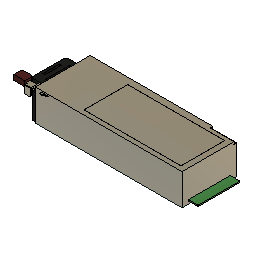
HPE flex psu (Autodesk Fusion 360 design; units mm, degrees)
Autodesk Fusion 360 part; units mm, degrees
sketch "Sketch1" plane through (0, 0, 0) normal (0, 0, 1) x (1, 0, 0)
  line L0 (-91.5, -34.15) -> (91.5, -34.15)
  line L1 (91.5, -34.15) -> (91.5, 34.15)
  line L2 (91.5, 34.15) -> (-91.5, 34.15)
  line L3 (-91.5, 34.15) -> (-91.5, -34.15)
  line L4 (-91.5, -34.15) -> (91.5, 34.15) construction
  line L5 (91.5, -34.15) -> (-91.5, 34.15) construction
  dimension "d1" = 183
  dimension "d2" = 68.3
  constraint horizontal L0
  constraint perpendicular L0 L1
  constraint parallel L0 L2
  constraint parallel L1 L3
  constraint coincident L4 origin
  constraint coincident L5 origin
  measures "d1" distance of L1.end L2.end
  measures "d2" distance of L0.end L1.end
extrude "Extrude1" add sketch "Sketch1" along normal blind 39.1 makes body 1
sketch "Sketch2" plane through (0, 0, 0) normal (0, 0, -1) x (1, 0, 0)
  line L0 (-91.5, 34.15) -> (-91.5, -34.15)
  line L1 (-91.5, -34.15) -> (91.5, -34.15)
  line L2 (91.5, -34.15) -> (91.5, 34.15)
  line L3 (91.5, 34.15) -> (-91.5, 34.15)
sketch "Sketch3" plane through (0, 34.15, 0) normal (0, 1, 0) x (-1, 0, 0)
  line L0 (-91.5, 0) -> (91.5, 0)
  line L1 (91.5, 0) -> (91.5, 39.1)
  line L2 (91.5, 39.1) -> (-91.5, 39.1)
  line L3 (-91.5, 39.1) -> (-91.5, 0)
  line L4 (91.5, 0) -> (91.5, 39.1)
  line L5 (61.5, 22.2) -> (121.5, 22.2)
  line L6 (121.5, 22.2) -> (121.5, 16.9)
  line L7 (121.5, 16.9) -> (61.5, 16.9)
  line L8 (61.5, 16.9) -> (61.5, 22.2)
  line L9 (61.5, 22.2) -> (121.5, 16.9) construction
  line L10 (121.5, 22.2) -> (61.5, 16.9) construction
  line L11 (82.2, 25.55) -> (100.8, 25.55)
  line L12 (100.8, 25.55) -> (100.8, 13.55)
  line L13 (100.8, 13.55) -> (82.2, 13.55)
  line L14 (82.2, 13.55) -> (82.2, 25.55)
  line L15 (82.2, 25.55) -> (100.8, 13.55) construction
  line L16 (100.8, 25.55) -> (82.2, 13.55) construction
  point P0 (91.5, 19.55)
  point P1 (91.5, 19.55)
  dimension "d5" = 60
  dimension "d6" = 5.3
  dimension "d7" = 18.6
  dimension "d8" = 12
  constraint coincident L0.end L1.start
  constraint coincident L1.end L2.start
  constraint horizontal L5
  constraint perpendicular L5 L6
  constraint parallel L5 L7
  constraint parallel L6 L8
  constraint coincident L9 P1
  constraint coincident L10 P1
  constraint midpoint L1 P1
  constraint horizontal L11
  constraint perpendicular L11 L12
  constraint parallel L11 L13
  constraint parallel L12 L14
  constraint coincident L15 P1
  constraint coincident L16 P1
  constraint coincident P1 P0
  measures "d5" distance of L6.end L7.end
  measures "d6" distance of L5.end L6.end
  measures "d7" distance of L12.end L13.end
  measures "d8" distance of L11.end L12.end
extrude "Extrude2" add sketch "Sketch3" against normal blind 43.7 contours L1 L4 L7 L12 L13 | L1 L4 L5 L7 L12 | L1 L4 L5 L11 L12 | L5 L6 L7 L12 bodies 1
sketch "Sketch4" plane through (0, 0, 16.9) normal (0, 0, -1) x (1, 0, 0)
  line L0 (-121.5, -34.15) -> (-100.8, -34.15)
  line L1 (-100.8, -34.15) -> (-100.8, 9.55)
  line L2 (-100.8, 9.55) -> (-121.5, 9.55)
  line L3 (-121.5, 9.55) -> (-121.5, -34.15)
  line L4 (-121.5, 9.55) -> (-100.8, 9.55)
  line L5 (-100.8, 9.55) -> (-100.8, -34.15)
  line L6 (-100.8, -34.15) -> (-121.5, -34.15)
  line L7 (-121.5, -34.15) -> (-121.5, 9.55)
  line L8 (-121.5, -7) -> (-110.5, -7)
  line L9 (-106.7103, 9.55) -> (-106.7103, 9)
  line L10 (-106.7103, 9) -> (-106.7103, 2.7)
  line L11 (-106.7103, 2.7) -> (-121.5, 2.7)
  line L12 (-110.5, -7) -> (-110.5, 2.7)
  line L13 (-106.7103, 2.7) -> (-86, 2.7)
  line L14 (-110.5, -7) -> (-110.5, -34.15)
  line L15 (-110.5, -34.15) -> (-110.5, -27.85)
  line L16 (-110.5, -27.85) -> (-100.8, -27.85)
  line L17 (-100.8, 2.7) -> (-100.8, -27.85)
  dimension "d11" = 11
  dimension "d12" = 6.3
  dimension "d13" = 6.3
  constraint horizontal L4
  constraint vertical L5
  constraint horizontal L6
  constraint vertical L7
  constraint coincident L0.end L1.start
  constraint coincident L2.end L3.start
  constraint coincident L3 L8.start
  constraint perpendicular L3 L8
  constraint coincident L2 L9.start
  constraint perpendicular L2 L9
  constraint perpendicular L4 L10
  constraint coincident L7 L11.end
  constraint perpendicular L7 L11
  constraint coincident L11 L12.end
  constraint perpendicular L11 L12
  constraint perpendicular L10 L13
  constraint coincident L6 L14.end
  constraint perpendicular L6 L14
  constraint parallel L14 L15
  constraint coincident L1 L16.end
  constraint perpendicular L1 L16
  constraint coincident L13 L17.start
  constraint coincident L5 L17.start
  measures "d11" distance of L8.start L8.end
  measures "d12" distance of L9.end L10.end
  measures "d13" distance of L14.end L15.end
extrude "Extrude3" cut sketch "Sketch4" against normal blind 45 contours L1 L5 L11 L12 L13 L14 L16 L17 bodies 1
sketch "Sketch5" plane through (0, 0, 13.55) normal (0, 0, -1) x (1, 0, 0)
  line L0 (-100.8, -34.15) -> (-91.5, -34.15)
  line L1 (-91.5, -34.15) -> (-91.5, 9.55)
  line L2 (-91.5, 9.55) -> (-100.8, 9.55)
  line L3 (-100.8, 9.55) -> (-100.8, -34.15)
  line L4 (-100.8, 9.55) -> (-91.5, -34.15)
  line L5 (-100.8, 5.2) -> (-91.5, 5.2)
  line L6 (-91.5, 5.2) -> (-91.5, -29.8)
  line L7 (-91.5, -29.8) -> (-100.8, -29.8)
  line L8 (-100.8, -29.8) -> (-100.8, 5.2)
  line L9 (-100.8, 5.2) -> (-91.5, -29.8) construction
  line L10 (-91.5, 5.2) -> (-100.8, -29.8) construction
  point P0 (-96.15, -12.3)
  dimension "d16" = 35
  constraint coincident L2.end L3.start
  constraint coincident L0.end L1.start
  constraint horizontal L5
  constraint perpendicular L5 L6
  constraint parallel L5 L7
  constraint parallel L6 L8
  constraint coincident L9 P0
  constraint coincident L10 P0
  constraint coincident L3 L5.start
  constraint midpoint L4 P0
  measures "d16" distance of L5.end L6.end
extrude "Extrude4" cut sketch "Sketch5" against normal blind 35 contours L3 L4 L5 L7 L8 | L1 L4 L5 L6 L7 bodies 1
sketch "Sketch6" plane through (0, 0, 16.9) normal (0, 0, -1) x (1, 0, 0)
  line L0 (-110.5, 2.7) -> (-100.8, 2.7)
  line L1 (-100.8, 2.7) -> (-100.8, 5.2)
  line L2 (-100.8, 5.2) -> (-100.8, 9.55)
  line L3 (-100.8, 9.55) -> (-121.5, 9.55)
  line L4 (-121.5, 9.55) -> (-121.5, -34.15)
  line L5 (-121.5, -34.15) -> (-100.8, -34.15)
  line L6 (-100.8, -34.15) -> (-100.8, -29.8)
  line L7 (-100.8, -29.8) -> (-100.8, -27.85)
  line L8 (-100.8, -27.85) -> (-110.5, -27.85)
  line L9 (-110.5, -27.85) -> (-110.5, 2.7)
  line L10 (-121.5, -2.463) -> (-118.3, -2.463)
  line L11 (-118.3, -2.463) -> (-118.3, -34.15)
  line L12 (-118.3, -2.463) -> (-118.3, 9.55)
  line L13 (-118.3, 9.55) -> (-118.3, -2.05)
  line L14 (-118.3, -34.15) -> (-118.3, -22.55)
  line L15 (-118.3, -2.05) -> (-115.7, -2.05)
  line L16 (-115.7, -2.05) -> (-118.3, -2.05)
  line L17 (-118.3, -2.05) -> (-118.3, -22.55)
  line L18 (-118.3, -22.55) -> (-115.7, -22.55)
  line L19 (-115.7, -22.55) -> (-115.7, -2.05)
  dimension "d19" = 3.2
  dimension "d20" = 11.6
  dimension "d21" = 11.6
  dimension "d22" = 2.6
  constraint coincident L4 L10.start
  constraint perpendicular L4 L10
  constraint coincident L5 L11.end
  constraint perpendicular L5 L11
  constraint coincident L3 L12.end
  constraint perpendicular L3 L12
  constraint perpendicular L3 L13
  constraint coincident L11 L14.end
  constraint perpendicular L13 L15
  constraint horizontal L16
  constraint vertical L17
  constraint horizontal L18
  constraint vertical L19
  measures "d19" distance of L10.start L10.end
  measures "d20" distance of L12.end L13.end
  measures "d21" distance of L11.end L14.end
  measures "d22" distance of L13.end L15.end
extrude "Extrude5" cut sketch "Sketch6" against normal blind 52 contours L11 L12 L15 L16 L17 L18 L19 bodies 1
sketch "Sketch7" plane through (-91.5, 0, 0) normal (-1, 0, 0) x (0, -1, 0)
  line L0 (-29.8, 13.55) -> (-34.15, 13.55)
  line L1 (-34.15, 13.55) -> (-34.15, 0)
  line L2 (-34.15, 0) -> (34.15, 0)
  line L3 (34.15, 0) -> (34.15, 39.1)
  line L4 (34.15, 39.1) -> (-34.15, 39.1)
  line L5 (-34.15, 39.1) -> (-34.15, 25.55)
  line L6 (-34.15, 25.55) -> (-29.8, 25.55)
  line L7 (-29.8, 25.55) -> (-29.8, 13.55)
  line L8 (5.2, 13.55) -> (5.2, 25.55)
  line L9 (5.2, 25.55) -> (9.55, 25.55)
  line L10 (9.55, 25.55) -> (9.55, 13.55)
  line L11 (9.55, 13.55) -> (5.2, 13.55)
  line L12 (34.15, 0) -> (34.15, 1.5)
  line L13 (34.15, 1.5) -> (10.35, 1.5)
  line L14 (10.35, 1.5) -> (10.35, 32.7)
  line L15 (10.35, 32.7) -> (34.15, 32.7)
  line L16 (34.15, 32.7) -> (34.15, 1.5)
  dimension "d25" = 1.5
  dimension "d26" = 23.8
  dimension "d27" = 31.2
  constraint coincident L2.end L3.start
  constraint perpendicular L2 L12
  constraint horizontal L13
  constraint vertical L14
  constraint horizontal L15
  constraint vertical L16
  measures "d25" distance of L2.end L12.end
  measures "d26" distance of L12.end L13.end
  measures "d27" distance of L12.end L15.end
extrude "Extrude6" add sketch "Sketch7" along normal blind 3.7 separate body contours L3 L13 L14 L15 L16 makes body 2
sketch "Sketch8" plane through (91.5, 0, 0) normal (1, 0, 0) x (0, 1, 0)
  line L0 (-34.15, 0) -> (34.15, 0)
  line L1 (34.15, 0) -> (34.15, 39.1)
  line L2 (34.15, 39.1) -> (-34.15, 39.1)
  line L3 (-34.15, 39.1) -> (-34.15, 0)
  line L4 (-34.15, 0) -> (34.15, 0)
  line L5 (34.15, 0) -> (34.15, 3.4)
  line L6 (34.15, 3.4) -> (-34.15, 3.4)
  line L7 (-34.15, 3.4) -> (-34.15, 0)
  line L8 (34.15, 3.4) -> (-34.15, 3.4)
  line L9 (-34.15, 3.4) -> (-34.15, 4.9)
  line L10 (-34.15, 4.9) -> (34.15, 4.9)
  line L11 (34.15, 4.9) -> (34.15, 3.4)
  line L12 (26.1, 3.4) -> (-26.1, 3.4)
  line L13 (-26.1, 3.4) -> (-26.1, 6.4)
  line L14 (-26.1, 6.4) -> (26.1, 6.4)
  line L15 (26.1, 6.4) -> (26.1, 3.4)
  line L16 (26.1, 3.4) -> (-26.1, 6.4) construction
  line L17 (-26.1, 3.4) -> (26.1, 6.4) construction
  point P0 (0, 4.9)
  dimension "d30" = 3.4
  dimension "d31" = 1.5
  dimension "d32" = 52.2
  constraint horizontal L4
  constraint vertical L5
  constraint horizontal L6
  constraint vertical L7
  constraint coincident L0.start L3.end
  constraint horizontal L8
  constraint vertical L9
  constraint horizontal L10
  constraint vertical L11
  constraint coincident L3 L9.end
  constraint horizontal L12
  constraint perpendicular L12 L13
  constraint parallel L12 L14
  constraint parallel L13 L15
  constraint coincident L16 P0
  constraint coincident L17 P0
  constraint coincident L6 L12.start
  constraint midpoint L10 P0
  measures "d30" distance of L0.start L6.end
  measures "d31" distance of L5.end L10.end
  measures "d32" distance of L13.end L14.end
extrude "Extrude7" add sketch "Sketch8" along normal blind 12 contours L6 L8 L10 L12 L13 L15 bodies 1
sketch "Sketch9" plane through (91.5, 0, 0) normal (1, 0, 0) x (0, 1, 0)
  line L0 (-26.1, 4.9) -> (26.1, 4.9)
  line L1 (26.1, 4.9) -> (26.1, 3.4)
  line L2 (26.1, 3.4) -> (-26.1, 3.4)
  line L3 (-26.1, 3.4) -> (-26.1, 4.9)
  line L4 (-34.15, 0) -> (34.15, 0)
  line L5 (34.15, 0) -> (34.15, 39.1)
  line L6 (34.15, 39.1) -> (-34.15, 39.1)
  line L7 (-34.15, 39.1) -> (-34.15, 0)
  line L8 (-34.15, 39.1) -> (-30.75, 39.1)
  line L9 (-30.75, 39.1) -> (-30.75, 36.1)
  line L10 (-30.75, 36.1) -> (-34.15, 36.1)
  line L11 (-34.15, 36.1) -> (-34.15, 39.1)
  dimension "d35" = 3.4
  dimension "d36" = 3
  constraint horizontal L8
  constraint vertical L9
  constraint horizontal L10
  constraint vertical L11
  constraint coincident L6.end L7.start
  measures "d35" distance of L6.end L8.end
  measures "d36" distance of L6.end L10.end
extrude "Extrude8" cut sketch "Sketch9" against normal blind 29.7 contours L6 L7 L8 L9 L10 L11 bodies 1
sketch "Sketch10" plane through (0, -34.15, 0) normal (0, -1, 0) x (1, 0, 0)
  line L0 (61.8, 36.1) -> (61.8, 39.1)
  line L1 (61.8, 39.1) -> (-91.5, 39.1)
  line L2 (-91.5, 39.1) -> (-91.5, 0)
  line L3 (-91.5, 0) -> (91.5, 0)
  line L4 (91.5, 0) -> (91.5, 36.1)
  line L5 (91.5, 36.1) -> (61.8, 36.1)
  line L6 (-91.5, 39.1) -> (-84.1, 39.1)
  line L7 (-84.1, 39.1) -> (-74.1, 39.1)
  line L8 (-84.1, 39.1) -> (-74.1, 39.1)
  line L9 (-74.1, 39.1) -> (-74.1, 36.3)
  line L10 (-74.1, 36.3) -> (-84.1, 36.3)
  line L11 (-84.1, 36.3) -> (-84.1, 39.1)
  line L12 (-74.1, 39.1) -> (-74.5, 39.1)
  line L13 (-74.1, 39.1) -> (-75.4, 39.1)
  line L14 (-75.4, 39.1) -> (-75.4, 36.5)
  line L15 (-75.4, 36.5) -> (-75.4, 36.3)
  line L16 (-75.4, 39.1) -> (-75.4, 37.4)
  line L17 (-75.4, 37.4) -> (-75.4, 36.4)
  line L18 (-75.4, 37.4) -> (-84.1, 37.4)
  line L19 (-84.1, 37.4) -> (-84.1, 36.4)
  line L20 (-84.1, 36.4) -> (-75.4, 36.4)
  line L21 (-75.4, 36.4) -> (-75.4, 37.4)
  dimension "d39" = 7.4
  dimension "d40" = 10
  dimension "d41" = 10
  dimension "d42" = 2.8
  dimension "d43" = 1.3
  dimension "d44" = 1.7
  dimension "d45" = 1
  dimension "d46" = 1
  constraint coincident L1.end L2.start
  constraint perpendicular L2 L6
  constraint perpendicular L2 L7
  constraint horizontal L8
  constraint vertical L9
  constraint horizontal L10
  constraint vertical L11
  constraint coincident L7 L12.end
  constraint perpendicular L9 L13
  constraint perpendicular L13 L14
  constraint coincident L10 L15.end
  constraint perpendicular L10 L15
  constraint perpendicular L13 L16
  constraint perpendicular L13 L17
  constraint horizontal L18
  constraint vertical L19
  constraint horizontal L20
  constraint vertical L21
  constraint coincident L11 L19.end
  measures "d39" distance of L1.end L6.end
  measures "d40" distance of L6.end L7.end
  measures "d41" distance of L6.end L7.end
  measures "d42" distance of L6.end L10.end
  measures "d43" distance of L7.end L13.end
  measures "d44" distance of L13.end L16.end
  measures "d45" distance of L16.end L17.end
  measures "d46" distance of L16.end L17.end
extrude "Extrude9" add sketch "Sketch10" along normal blind 2.2 contours L11 L14 L15 L17 L18 L19 L20 L21 bodies 1
sketch "Sketch11" plane through (0, 0, 37.4) normal (0, 0, 1) x (-1, 0, 0)
  line L0 (75.4, 34.15) -> (84.1, 34.15)
  line L1 (84.1, 34.15) -> (84.1, 36.35)
  line L2 (84.1, 36.35) -> (75.4, 36.35)
  line L3 (75.4, 36.35) -> (75.4, 34.15)
  line L4 (84.1, 36.35) -> (81.7, 36.35)
  line L5 (81.7, 36.35) -> (75.4, 34.15)
  dimension "d49" = 2.4
  constraint coincident L1.end L2.start
  constraint perpendicular L1 L4
  constraint coincident L0.start L3.end
  measures "d49" distance of L1.end L4.end
extrude "Extrude10" cut sketch "Sketch11" against normal blind 3 contours L2 L3 L5 bodies 1
extrude "Extrude11" add 1 faces at (-84.1, -35.6167, 36.7333) along direction (-1, 0, 0) blind 7.4 separate body on bodies 1 makes body 3
extrude "Extrude12" add 1 faces at (-91.5, -35.6167, 36.7333) along direction (-1, 0, 0) blind 3.3 separate body on bodies 3 makes body 4
extrude "Extrude13" add 1 faces at (-93.7, -34.15, 36.7333) along direction (0, 1, 0) blind 9.2 separate body on bodies 4 makes body 5
extrude "Extrude14" add 1 faces at (-94.8, -31.0833, 36.7333) along direction (-1, 0, 0) blind 1 separate body on bodies 5 makes body 6
extrude "Extrude15" add 1 faces at (-95.1333, -31.0833, 36.4) along direction (0, 0, -1) blind 2.6 on bodies 6 bodies 4 6 5
extrude "Extrude16" add 1 faces at (-95.1333, -31.0833, 33.8) along direction (0, 0, -1) blind 1 separate body on bodies 4 makes body 7
extrude "Extrude17" add 1 faces at (-95.8, -31.0833, 33.4667) along direction (-1, 0, 0) blind 25.4 on bodies 7 bodies 4 7
extrude "Extrude18" cut 1 faces at (-94.8, -35.6167, 36.7333) along direction (1, 0, 0) blind 4 on bodies 4 bodies 3 4
delete_body "RemoveBody1" bodies 3
sketch "Sketch12" plane through (0, 0, 33.8) normal (0, 0, 1) x (-1, 0, 0)
  line L0 (95.8, 34.15) -> (95.8, 24.95)
  line L1 (95.8, 24.95) -> (121.2, 24.95)
  line L2 (121.2, 24.95) -> (121.2, 34.15)
  line L3 (121.2, 34.15) -> (95.8, 34.15)
  line L4 (95.8, 34.15) -> (97.8, 34.15)
  line L5 (97.8, 34.15) -> (97.8, 24.95)
  line L6 (97.8, 24.95) -> (97.8, 31.45)
  line L7 (97.8, 31.45) -> (121.2, 31.45)
  line L8 (97.8, 24.95) -> (97.8, 29.55)
  line L9 (97.8, 29.55) -> (121.2, 29.55)
  line L10 (97.8, 31.45) -> (106.1, 31.45)
  line L11 (97.8, 31.45) -> (99.1, 31.45)
  line L12 (99.1, 31.45) -> (106.1, 31.45)
  line L13 (106.1, 31.45) -> (106.1, 34.15)
  line L14 (106.1, 34.15) -> (99.1, 34.15)
  line L15 (99.1, 34.15) -> (99.1, 31.45)
  line L16 (97.8, 34.15) -> (99.1, 34.15)
  line L17 (99.1, 34.15) -> (99.1, 31.45)
  line L18 (99.1, 31.45) -> (97.8, 31.45)
  line L19 (97.8, 31.45) -> (97.8, 34.15)
  line L20 (106.1, 34.15) -> (121.2, 34.15)
  line L21 (121.2, 34.15) -> (121.2, 29.55)
  line L22 (121.2, 29.55) -> (106.1, 29.55)
  line L23 (106.1, 29.55) -> (106.1, 34.15)
  line L24 (97.8, 24.95) -> (97.8, 32.95)
  line L25 (97.8, 32.95) -> (99.1, 32.95)
  line L26 (99.1, 32.95) -> (106.1, 32.95)
  line L27 (106.1, 32.95) -> (106.1, 31.95)
  line L28 (106.1, 31.95) -> (99.1, 31.95)
  line L29 (99.1, 31.95) -> (99.1, 32.95)
  dimension "d68" = 2
  dimension "d69" = 6.5
  dimension "d70" = 4.6
  dimension "d71" = 8.3
  dimension "d72" = 1.3
  dimension "d73" = 8
  dimension "d74" = 1
  constraint coincident L0.start L3.end
  constraint perpendicular L0 L4
  constraint coincident L1 L5.end
  constraint perpendicular L1 L5
  constraint perpendicular L1 L6
  constraint coincident L2 L7.end
  constraint perpendicular L2 L7
  constraint perpendicular L1 L8
  constraint midpoint L2 L9.end
  constraint perpendicular L5 L10
  constraint perpendicular L5 L11
  constraint horizontal L12
  constraint vertical L13
  constraint horizontal L14
  constraint vertical L15
  constraint coincident L3 L13.end
  constraint horizontal L16
  constraint vertical L17
  constraint horizontal L18
  constraint vertical L19
  constraint horizontal L20
  constraint vertical L21
  constraint horizontal L22
  constraint vertical L23
  constraint coincident L8 L5.end
  constraint perpendicular L1 L24
  constraint coincident L17 L25.end
  constraint perpendicular L17 L25
  constraint horizontal L26
  constraint vertical L27
  constraint horizontal L28
  constraint vertical L29
  measures "d68" distance of L0.start L4.end
  measures "d69" distance of L5.end L6.end
  measures "d70" distance of L5.end L8.end
  measures "d71" distance of L6.end L10.end
  measures "d72" distance of L6.end L11.end
  measures "d73" distance of L5.end L24.end
  measures "d74" distance of L25.end L28.end
extrude "Extrude19" add sketch "Sketch12" against normal blind 10 contours L13 L15 L17 L23 L26 L27 L28 L29 bodies 4
extrude "Extrude20" cut sketch "Sketch12" against normal blind 3 contours L3 L5 L15 L16 L17 L19 L25 | L3 L13 L14 L15 L17 L23 L26 | L5 L7 L10 L11 L15 L17 L18 L19 L24 L25 L29 | L2 L3 L7 L13 L20 L21 L23 L27 | L2 L7 L9 L21 L22 L23 bodies 4
sketch "Sketch13" plane through (0, 0, 33.8) normal (0, 0, 1) x (-1, 0, 0)
  line L0 (121.2, 29.55) -> (106.1, 29.55)
  line L1 (106.1, 29.55) -> (106.1, 32.95)
  line L2 (106.1, 32.95) -> (99.1, 32.95)
  line L3 (99.1, 32.95) -> (99.1, 31.45)
  line L4 (99.1, 31.45) -> (97.8, 31.45)
  line L5 (97.8, 31.45) -> (97.8, 34.15)
  line L6 (97.8, 34.15) -> (95.8, 34.15)
  line L7 (95.8, 34.15) -> (95.8, 24.95)
  line L8 (95.8, 24.95) -> (121.2, 24.95)
  line L9 (121.2, 24.95) -> (121.2, 29.55)
  line L10 (121.2, 29.55) -> (107.5, 29.55)
  line L11 (107.5, 29.55) -> (121.2, 24.95)
  line L12 (121.2, 24.95) -> (107.5, 24.95)
  line L13 (107.5, 24.95) -> (107.5, 29.55)
  line L14 (107.5, 29.55) -> (121.2, 29.55)
  line L15 (121.2, 29.55) -> (121.2, 24.95)
  line L16 (121.2, 24.95) -> (107.5, 29.55) construction
  line L17 (107.5, 24.95) -> (121.2, 29.55) construction
  line L18 (121.2, 24.95) -> (107.5, 24.95)
  line L19 (107.5, 24.95) -> (107.5, 21.15)
  line L20 (107.5, 21.15) -> (121.2, 21.15)
  line L21 (121.2, 21.15) -> (121.2, 24.95)
  line L22 (121.2, 21.15) -> (107.5, 21.15)
  line L23 (107.5, 21.15) -> (107.5, 31.45)
  line L24 (107.5, 31.45) -> (121.2, 31.45)
  line L25 (121.2, 31.45) -> (121.2, 21.15)
  point P0 (114.35, 27.25)
  dimension "d79" = 13.7
  dimension "d80" = 13.7
  dimension "d81" = 3.8
  dimension "d82" = 10.3
  constraint coincident L0.start L9.end
  constraint perpendicular L9 L10
  constraint coincident L8.end L9.start
  constraint horizontal L12
  constraint perpendicular L12 L13
  constraint parallel L12 L14
  constraint parallel L13 L15
  constraint coincident L16 P0
  constraint coincident L17 P0
  constraint midpoint L11 P0
  constraint horizontal L18
  constraint vertical L19
  constraint horizontal L20
  constraint vertical L21
  constraint horizontal L22
  constraint vertical L23
  constraint horizontal L24
  constraint vertical L25
  measures "d79" distance of L0.start L10.end
  measures "d80" distance of L8.end L12.end
  measures "d81" distance of L8.end L20.end
  measures "d82" distance of L20.end L24.end
extrude "Extrude21" add sketch "Sketch13" along normal blind 2.75 separate body contours L0 L10 L14 L23 L24 L25 | L8 L12 L18 L19 L20 L21 L22 L23 L25 makes body 8 at (-112.0667, -31.45, 34.7167) makes body 9 at (-116.6333, -22.4167, 33.8)
extrude "Extrude22" add 2 faces at (-112.0667, -30.8167, 33.8) (-116.6333, -22.4167, 33.8) along direction (0, 0, -1) blind 3.75 on bodies 8 9 bodies 4 8 9
extrude "Extrude23" add 2 faces at (-112.0667, -24.95, 31.8833) (-116.6333, -24.95, 34.7167) along direction (0, -1, 0) blind 6.5 on bodies 4 bodies 4
chamfer "Chamfer1" distance 2 angle 45 2 edges at (-121.2, -21.15, 33.3) (-107.5, -21.15, 33.3) on bodies 4
chamfer "Chamfer2" distance 2 angle 45 2 edges at (-121.5, 34.15, 19.55) (-121.5, -9.55, 19.55) on bodies 1
fillet "Fillet1" radius 0.5 6 edges at (-95.8, -29.55, 37.4) (-94.8, -29.55, 36.4) (-94.8, -29.55, 32.8) (-95.8, -29.55, 33.8) (-102.6, -32.95, 33.8) (-102.6, -31.95, 32.8) on bodies 4
fillet "Fillet2" radius 1 2 edges at (-99.1, -32.45, 23.8) (-106.1, -32.45, 23.8) on bodies 4
chamfer "Chamfer3" distance 1 angle 45 2 edges at (103.5, -26.1, 4.15) (103.5, 26.1, 4.15) on bodies 1
mirror "Mirror1" about plane through (0, 0, 0) normal (0, 1, 0) of "Extrude8"
extrude "Extrude24" add 1 faces at (81.6, -31.8833, 36.1) along direction (0, 0, 1) blind 3 on bodies 1 bodies 1
sketch "Sketch14" plane through (0, 0, 39.1) normal (0, 0, 1) x (-1, 0, 0)
  line L0 (-91.5, -30.75) -> (-61.8, -30.75)
  line L1 (-61.8, -30.75) -> (-61.8, -34.15)
  line L2 (-61.8, -34.15) -> (91.5, -34.15)
  line L3 (91.5, -34.15) -> (91.5, 34.15)
  line L4 (91.5, 34.15) -> (-91.5, 34.15)
  line L5 (-91.5, 34.15) -> (-91.5, -30.75)
  line L6 (-91.5, 26.4218) -> (-84.4, 26.4218)
  line L7 (-81.1016, 34.15) -> (-81.1016, 28.45)
  line L8 (-81.1016, 28.45) -> (-84.468, 28.45)
  line L9 (-84.468, 28.45) -> (-84.468, 26.4218)
  line L10 (-84.468, 26.4218) -> (-81.1016, 26.4218)
  line L11 (-81.1016, 26.4218) -> (-81.1016, 28.45)
  line L12 (-84.468, 28.45) -> (36.532, 28.45)
  line L13 (36.532, 28.45) -> (36.532, -26.15)
  line L14 (36.532, -26.15) -> (-84.468, -26.15)
  line L15 (-84.468, -26.15) -> (-84.468, 28.45)
  line L16 (36.532, -26.15) -> (32.732, -26.15)
  line L17 (32.732, -26.15) -> (32.732, -23.55)
  line L18 (32.732, -23.55) -> (36.532, -23.55)
  line L19 (36.532, -23.55) -> (36.532, -26.15)
  line L20 (32.732, -23.55) -> (-76.768, -23.55)
  line L21 (-76.768, -23.55) -> (-76.768, 26.35)
  line L22 (-76.768, 26.35) -> (32.732, 26.35)
  line L23 (32.732, 26.35) -> (32.732, -23.55)
  dimension "d100" = 7.1
  dimension "d101" = 5.7
  dimension "d102" = 121
  dimension "d103" = 54.6
  dimension "d104" = 3.8
  dimension "d105" = 2.6
  dimension "d106" = 109.5
  dimension "d107" = 49.9
  constraint coincident L5 L6.start
  constraint perpendicular L5 L6
  constraint coincident L4 L7.start
  constraint perpendicular L4 L7
  constraint horizontal L8
  constraint vertical L9
  constraint horizontal L10
  constraint vertical L11
  constraint coincident L6 L9.end
  constraint horizontal L12
  constraint vertical L13
  constraint horizontal L14
  constraint vertical L15
  constraint horizontal L16
  constraint vertical L17
  constraint horizontal L18
  constraint vertical L19
  constraint horizontal L20
  constraint vertical L21
  constraint horizontal L22
  constraint vertical L23
  measures "d100" distance of L6.start L6.end
  measures "d101" distance of L7.start L7.end
  measures "d102" distance of L8.end L12.end
  measures "d103" distance of L8.end L14.end
  measures "d104" distance of L13.end L16.end
  measures "d105" distance of L13.end L18.end
  measures "d106" distance of L17.end L20.end
  measures "d107" distance of L17.end L22.end
extrude "Extrude25" cut sketch "Sketch14" against normal blind 0.15 contours L20 L21 L22 L23 bodies 1
extrude "Extrude26" cut sketch "Sketch14" against normal blind 0.1 contours L6 L8 L9 L10 L11 L12 L15 | L6 L10 L11 L12 L13 L14 L15 L17 L18 | L13 L14 L16 L17 L18 L19 bodies 1
copy_body "Body->Comp1" bodies 4 removing the originals makes body 10 in component "Component"
copy_body "Body->Comp2" bodies 2 removing the originals makes body 11 in component "Component'"
copy_body "Body->Comp3" bodies 1 removing the originals makes body 12 in component "Component''"
split "Split1" by plane through (-91.5, 34.15, 0) normal (-1, 0, 0) bodies 12 makes body 13 at (-110.2667, -7.2667, 22.2) in component "Component''"
delete_face "DeleteFace1" 1 faces at (3.768, 6.9167, 38.95) on bodies 12 in component "Component''"
extrude "Extrude1'" add 1 faces at (3.768, 23.55, 26) along direction (0, -1, 0) blind 57.7 on bodies 12 bodies 12 in component "Component''"
component "Component" placed x (1, 0, 0) y (0, 1, 0) z (0, 0, 1) at (0, 0, 0)
component "Component'" placed x (1, 0, 0) y (0, 1, 0) z (0, 0, 1) at (0, 0, 0)
component "Component''" placed x (1, 0, 0) y (0, 1, 0) z (0, 0, 1) at (0, 0, 0)
equation "d7 = ( 9.3 * 2 ) * 1 mm"
equation "d60 = 4.6 mm - 2 mm"
equation "d71 = 7 mm + 1.3 mm"
equation "d85 = 1 mm + 2.75 mm"
